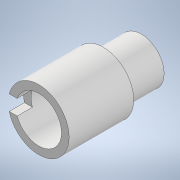
# Autodesk Inventor part: handle_base3
Saved by Autodesk Inventor 2021 (Build 250183000, 183)
## iProperties
Created: 2021-07-05
Part Number: handle_base3
Material: Generic
Document SubType Name: Modeling
Designer: teh18
Density: 1 g/cm^3
Appearance: Default
Author: teh18
Autodesk Inventor part; units mm, degrees
ref_plane "YZ Plane" through (0, 0, 0) normal (1, 0, 0) x (0, 1, 0)
ref_plane "XZ Plane" through (0, 0, 0) normal (0, 1, 0) x (-1, 0, 0)
ref_plane "XY Plane" through (0, 0, 0) normal (0, 0, 1) x (1, 0, 0)
sketch "Sketch1" plane through (0, 0, 0) normal (0, 0, 1) x (1, 0, 0)
  circle A0 centre (0, 0) radius 6.1 projected
  circle A1 centre (0, 0) radius 8 projected
  circle A2 centre (0.0908, 0.2329) radius 5 projected
  circle A3 centre (0, 0) radius 6.1 projected
  circle A4 centre (0, 0) radius 6
  point P0 (0, 0)
  dimension "d0" = 0.1
  constraints: 1 centre point
  measures "d0" radial gap between concentric circles of A0 A4
extrude "Extrusion1" add sketch "Sketch1" against normal blind 10 contours A4
sketch "Sketch2" plane through (0, 0, 0) normal (0, 0, 1) x (1, 0, 0)
  circle A0 centre (0, 0) radius 6.1 projected
  circle A1 centre (0, 0) radius 8 projected
  circle A2 centre (0, 0) radius 6 projected
  point P0 (0, 0)
extrude "Extrusion2" add sketch "Sketch2" along normal blind 17 contours A0 | A1
sketch "Sketch3" plane through (0, 0, 17) normal (0, 0, 1) x (1, 0, 0)
  line L0 (-1.3404, -2) -> (-8, -2)
  line L1 (-8, -2) -> (-8, 2)
  line L2 (-8, 2) -> (-1.3404, 2)
  line L3 (-1.3404, 2) -> (-1.3404, -2)
  line L4 (-1.3404, -2) -> (-8, 2) construction
  line L5 (-8, -2) -> (-1.3404, 2) construction
  point P0 (0, 0)
  point P1 (-4.6702, 0)
  dimension "d5" = 4
  constraints: 12 end point, 2 midpoint, 2 parallel, 1 horizontal, 1 perpendicular
  measures "d5" distance of L0.end L1.end
extrude "Extrusion3" cut sketch "Sketch3" against normal blind 4
body "Solid1"
